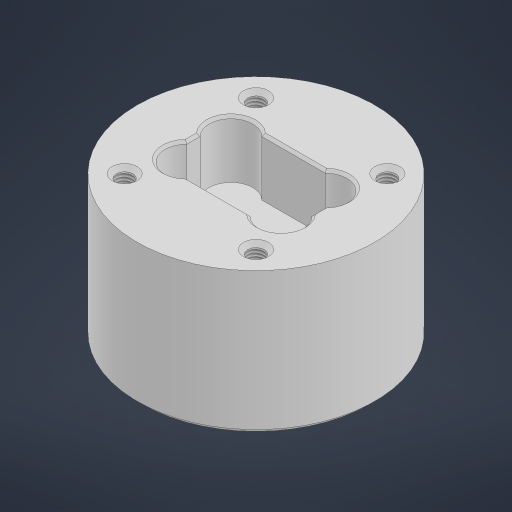
# Autodesk Inventor part: HM1_FIXT1-001
Saved by Autodesk Inventor 2024.3 (Build 283343000, 343)
## iProperties
Created: 2024-08-19
Part Number: HM1_FIXT1-001
Material: Generic
Document SubType Name: Modeling
Designer: fablabadmin
Density: 1 g/cm^3
Appearance: Default
holeL: 52,500 mm
Author: fablabadmin
Autodesk Inventor part; units mm, degrees
ref_plane "YZ Plane" through (0, 0, 0) normal (1, 0, 0) x (0, 1, 0)
ref_plane "XZ Plane" through (0, 0, 0) normal (0, 1, 0) x (-1, 0, 0)
ref_plane "XY Plane" through (0, 0, 0) normal (0, 0, 1) x (1, 0, 0)
sketch "Sketch1" plane through (0, 0, 0) normal (0, 1, 0) x (-1, 0, 0)
  circle A0 centre (0, 0) radius 47.5
  line L0 (-25, 15) -> (25, 15)
  line L1 (25, 15) -> (25, -15)
  line L2 (25, -15) -> (-25, -15)
  line L3 (-25, -15) -> (-25, 15)
  line L4 (-25, 15) -> (25, -15) construction
  line L5 (25, 15) -> (-25, -15) construction
  line L6 (-26.25, 26.25) -> (26.25, 26.25) construction
  line L7 (26.25, 26.25) -> (26.25, -26.25) construction
  line L8 (26.25, -26.25) -> (-26.25, -26.25) construction
  line L9 (-26.25, -26.25) -> (-26.25, 26.25) construction
  line L10 (-26.25, 26.25) -> (26.25, -26.25) construction
  line L11 (26.25, 26.25) -> (-26.25, -26.25) construction
  dimension "d0" = 30
  dimension "d2" = 95
  dimension "holeL" = 52.5
  dimension "d27" = 50
  constraints: 32 end point, 5 coincident, 4 midpoint, 4 parallel, 3 perpendicular, 2 horizontal, 1 centre point
  measures "d0" distance of L2.end L0.start
  measures "d2" diameter of A0
  measures "holeL" distance of L8.end L6.start
  measures "d27" distance between parallel lines of L3 L1
extrude "Extrusion1" add sketch "Sketch1" against normal blind 57 contours A0 | L0 L1 L2 L3
extrude "Extrusion2" cut sketch "Sketch1" against normal blind 23 contours L0 L1 L2 L3
sketch "Sketch3" plane through (0, 0, 0) normal (0, 1, 0) x (1, 0, 0)
  line L0 (-25, -15) -> (-25, 15) construction
  line L1 (-25, 15) -> (25, 15) construction
  line L2 (25, 15) -> (25, -15) construction
  line L3 (25, -15) -> (-25, -15) construction
  circle A0 centre (0, 0) radius 47.5 construction
  circle A1 centre (18.8128, 8.8128) radius 8.75
  line L4 (18.8128, 8.8128) -> (25, 15) construction
  line L5 (-66.5, 0) -> (66.5, 0) construction
  line L6 (0, 66.5) -> (0, -66.5) construction
  circle A2 centre (18.8128, -8.8128) radius 8.75
  circle A3 centre (-18.8128, 8.8128) radius 8.75
  circle A4 centre (-18.8128, -8.8128) radius 8.75
  dimension "d34" = 17.5
  dimension "d33" = 45
  constraints: 3 centre point, 3 symmetric about line, 2 end point, 6 other
  measures "d33" angle of L2 L4
extrude "Extrusion3" cut sketch "Sketch3" against normal up to surface (23 mm away)
hole "Hole1" at (-26.25, 0, -26.25) at (26.25, 0, -26.25) at (26.25, 0, 26.25) at (-26.25, 0, 26.25) direction (0, -1, 0) diameter 6.647 depth 17 tip angle 118 countersink diameter 10 countersink angle 90 thread size "M8x1.25" class "6H" standard "ISO Metric profile"
chamfer "Chamfer1" distance 1 angle 45 8 edges at (0, 0, -15) (25, 0, 0) (0, 0, 15) (-25, 0, 0) (-25, 0, -15) (-25, 0, 15) (25, 0, -15) (25, 0, 15)
chamfer "Chamfer2" distance 2 angle 45 1 edges at (47.5, -57, 0)
sketch "Sketch2" plane through (0, -57, 0) normal (0, -1, 0) x (1, 0, 0)
  circle A0 centre (0, 0) radius 15 construction
  circle A1 centre (0, 0) radius 19 construction
  dimension "d23" = 4
  dimension "d24" = 30
  constraints: 2 centre point, 2 coincident, 2 other
  measures "d23" radial gap between concentric circles of A0 A1
  measures "d24" diameter of A0
mark "Mark1"
body "Solid1"
